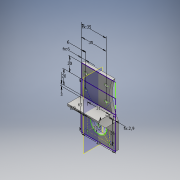
# Autodesk Inventor part: support_nema17_40mm
Saved by Autodesk Inventor 2016 (Build 200138000, 138)
## iProperties
Created: 2018-01-08
Part Number: support_nema17_40mm
Material: Generic
Document SubType Name: Modeling
Designer: mbouhier
Density: 1 g/cm^3
Appearance: Default
Author: mbouhier
Autodesk Inventor part; units mm, degrees
ref_plane "YZ Plane" through (0, 0, 0) normal (1, 0, 0) x (0, 1, 0)
ref_plane "XZ Plane" through (0, 0, 0) normal (0, 1, 0) x (-1, 0, 0)
ref_plane "XY Plane" through (0, 0, 0) normal (0, 0, 1) x (1, 0, 0)
sketch "Sketch1" plane through (0, 0, 0) normal (0, 1, 0) x (-1, 0, 0)
  line L0 (-24, 32.5) -> (24, 32.5)
  line L1 (24, 32.5) -> (24, -32.5)
  line L2 (24, -32.5) -> (-24, -32.5)
  line L3 (-24, -32.5) -> (-24, 32.5)
  line L4 (-24, 32.5) -> (24, -32.5) construction
  line L5 (24, 32.5) -> (-24, -32.5) construction
  line L6 (24, 9.5) -> (-24, 9.5)
  line L7 (-24, 9.5) -> (-24, -32.5)
  line L8 (-24, -32.5) -> (24, -32.5)
  line L9 (24, -32.5) -> (24, 9.5)
  circle A0 centre (0, -11.5) radius 11.25
  line L10 (24, 12.5) -> (-24, 12.5)
  line L11 (-24, 24.95) -> (-24, 20.05)
  line L12 (15.5, -27) -> (-15.5, -27) construction
  line L13 (-15.5, -27) -> (-15.5, 4) construction
  line L14 (-15.5, 4) -> (15.5, 4) construction
  line L15 (15.5, 4) -> (15.5, -27) construction
  line L16 (15.5, -27) -> (-15.5, 4) construction
  line L17 (-15.5, -27) -> (15.5, 4) construction
  line L18 (-24, 52.5) -> (24, 52.5)
  line L19 (24, 52.5) -> (24, 32.5)
  line L20 (24, 32.5) -> (-24, 32.5)
  line L21 (-24, 32.5) -> (-24, 52.5)
  point P0 (0, 0)
  point P1 (-21.1, 9.5)
  point P2 (21.1, 9.5)
  point P3 (18, 42.6936)
  point P4 (-11, 42.5)
  point P5 (18, 22.5)
  point P6 (-11, 22.3064)
  dimension "d0" = 48
  dimension "d1" = 65
  dimension "d2" = 20
  dimension "d3" = 3
  dimension "d4" = 2.9
  dimension "d5" = 2.9
  dimension "d6" = 22.5
  dimension "d35" = 31
  dimension "d36" = 31
  dimension "d71" = 20
  dimension "d73" = 6
  dimension "d74" = 6
  dimension "d82" = 35
  dimension "d83" = 35
  constraints: 44 end point, 8 parallel, 6 point on line, 5 coincident, 5 perpendicular, 4 horizontal, 4 midpoint, 1 centre point
  measures "d0" distance of L1.end L2.end
  measures "d1" distance of L0.end L1.end
  measures "d2" distance from line of L10.start L0
  measures "d3" distance of L6.start L10.start
  measures "d4" distance from line of L1 point (21.1, 9.5)
  measures "d5" distance from line of L3 point (-21.1, 9.5)
  measures "d6" diameter of A0
  measures "d35" distance of L13.end L14.end
  measures "d36" distance of L12.end L13.end
  measures "d71" distance between parallel lines of L18 L0
  measures "d73" distance from line of L1 point (18, 22.5)
  measures "d74" distance from line of L19 point (18, 42.694)
  measures "d82" distance from line of point (-11, 42.5) L19
  measures "d83" distance from line of L1 point (-11, 22.306)
extrude "Extrusion1" add sketch "Sketch1" along normal blind 4.2
sketch "Sketch2" plane through (0, 4.2, 0) normal (0, 1, 0) x (1, 0, 0)
  point P0 (0, 0)
  point P1 (11, -42.5)
  point P2 (11, -22.3064)
  point P3 (-18, -22.5)
  point P4 (-18, -42.6936)
hole "Hole5" at (11, 4.2, 42.5) at (-18, 4.2, 42.6936) at (11, 4.2, 22.3064) at (-18, 4.2, 22.5) direction (0, -1, 0) diameter 4.5 end through all
extrude "Extrusion3" add sketch "Sketch1" against normal blind 20 contours L1 L6 L3 L10
sketch "Sketch4" plane through (24, 0, -32.5) normal (1, 0, 0) x (0, 0, -1)
  line L0 (-42, -20) -> (-42, 0) projected
  line L1 (-42, -20) -> (-22, 0)
  line L2 (0, 0) -> (-42, 0) projected
  line L3 (-22, 0) -> (-42, 0)
  line L4 (-42, 0) -> (-42, -20)
  point P0 (-32.5, 0)
  dimension "d32" = 20
  constraints: 6 end point, 2 collinear
  measures "d32" distance from line of L1.end L0
extrude "Extrusion4" add sketch "Sketch4" against normal blind 2.7
ref_plane "Work Plane1" through (0, 0, 52.5) normal (-1, 0, 0) x (0, 0, 1)
mirror "Mirror1" about plane through (0, 0, 52.5) normal (-1, 0, 0) of "Extrusion4"
sketch "Sketch5" plane through (0, 4.2, 0) normal (0, 1, 0) x (1, 0, 0)
  point P0 (0, 0)
  point P1 (-15.5, 27)
  point P2 (15.5, 27)
  point P3 (-15.5, -4)
  point P4 (15.5, -4)
hole "Hole4" at (-15.5, 4.2, -27) at (15.5, 4.2, -27) at (-15.5, 4.2, 4) at (15.5, 4.2, 4) direction (0, -1, 0) diameter 3.2 depth 8 tip angle 118 countersink diameter 6 countersink angle 90
sketch "Sketch6" plane through (21.3, -20, 9.5) normal (0, 0, -1) x (-1, 0, 0)
  line L0 (42.6, 0) -> (42.6, 20) projected
  line L1 (0, 20) -> (42.6, 20) projected
  line L2 (0, 20) -> (0, 0) projected
  line L3 (42.6, 0) -> (0, 0) projected
  point P0 (21.3, 20)
extrude "ajustement 0.2mm" cut sketch "Sketch6" against normal blind 0.4
sketch "Sketch7" plane through (0, 4.2, 0) normal (0, 1, 0) x (1, 0, 0)
  circle A0 centre (70.6822, -32.5) radius 55
  line L0 (21.3, -9.9) -> (-21.3, -9.9) construction
  line L1 (21.3, -9.9) -> (21.3, -51.2) construction
  line L2 (137, -22.5) -> (-72, -22.5) construction
  line L3 (0, -123.9517) -> (0, 131.2102) construction
  circle A1 centre (0, 11.5) radius 83.2585 construction
  line L4 (134.8387, -42.5) -> (-75.1613, -42.5) construction
  line L5 (134.8387, -32.5) -> (-75.1613, -32.5) construction
  point P0 (0, 0)
  dimension "d67" = 166.517
  dimension "d53" = 110
  dimension "d69" = 20
  dimension "d70" = 10
  constraints: 8 end point, 3 horizontal, 2 coincident, 1 centre point, 1 point on line, 1 vertical, 3 other
  measures "d53" diameter of A0
  measures "d69" distance between parallel lines of L4 L2
  measures "d70" distance between parallel lines of L5 L2
sketch "Sketch8" plane through (0, 0, 0) normal (0, -1, 0) x (1, 0, 0)
  line L0 (-21.3, 9.9) -> (21.3, 9.9) projected
  line L1 (21.3, -10.5) -> (21.3, 9.5) projected
  line L2 (-21.3, -10.5) -> (-21.3, 9.5) projected
  line L3 (21.3, 9.9) -> (-21.3, 9.9) projected
  line L4 (-18.3, 9.9) -> (-21.3, 6.9)
  line L5 (-21.3, 9.9) -> (-21.3, -10.5) projected
  line L6 (18.3, 9.9) -> (21.3, 6.9)
  line L7 (21.3, -10.5) -> (21.3, 9.9) projected
  point P0 (0, 0)
  dimension "d54" = 3
  dimension "d55" = 3
  dimension "d56" = 3
  dimension "d57" = 3
  constraints: 4 end point, 4 point on line
  measures "d54" distance from line of L2 L4.start
  measures "d55" distance from line of L4.end L0
  measures "d56" distance from line of L6.start L1
  measures "d57" distance from line of L6.end L0
extrude "Extrusion6" add sketch "Sketch8" along normal blind 20
sketch "Sketch9" plane through (24, 0, -32.5) normal (1, 0, 0) x (0, 0, -1)
  line L0 (-39.4, -20) -> (-42, -20) projected
  line L1 (-39.4, -17.4) -> (-39.4, -20) projected
  line L2 (-42, -20) -> (-22, 0) projected
  point P0 (-32.5, 0)
extrude "Extrusion7" cut sketch "Sketch9" against normal through all
extrude "Extrusion8" cut sketch "Sketch7" against normal blind 30
sketch "Sketch10" plane through (-24, -20, 12.5) normal (0, 0, 1) x (1, 0, 0)
  line L0 (43.4475, 0) -> (43.4475, 20) projected
  line L1 (0, 20) -> (43.4475, 20) projected
  line L2 (0, 20) -> (0, 0) projected
  line L3 (43.4475, 0) -> (0, 0) projected
  point P0 (24, 20)
extrude "ajustement 0.2" cut sketch "Sketch10" against normal blind 0.2
equation "\"d5\" = d4"
equation "\"d74\" = d73"
equation "\"d83\" = d82"
equation "\"d55\" = d54"
equation "\"d56\" = d54"
equation "\"d57\" = d56"
body "Solid1"
